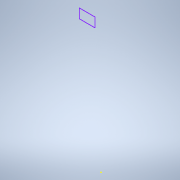
# Autodesk Inventor part: meios
Saved by Autodesk Inventor 2020 (Build 240168000, 168)
## iProperties
Created: 2020-04-25
Part Number: meios
Material: Genérico
Document SubType Name: Modeling
Designer: gi-se
Density: 1 g/cm^3
Appearance: Padrão
Author: gi-se
Autodesk Inventor part; units mm, degrees
ref_plane "YZ Plane" through (0, 0, 0) normal (1, 0, 0) x (0, 1, 0)
ref_plane "XZ Plane" through (0, 0, 0) normal (0, 1, 0) x (-1, 0, 0)
ref_plane "XY Plane" through (0, 0, 0) normal (0, 0, 1) x (1, 0, 0)
sketch "Esboço1" plane through (0, 0, 0) normal (0, 0, 1) x (1, 0, 0)
  line L0 (-7, 39) -> (-2, 39)
  line L1 (-2, 39) -> (-2, 42)
  line L2 (-2, 42) -> (-7, 42)
  line L3 (-7, 42) -> (-7, 39)
  point P0 (0, 0)
  constraints: 8 end point, 2 parallel, 1 horizontal, 1 perpendicular
extrude "Extrusão1" add sketch "Esboço1" along normal blind 66.1
